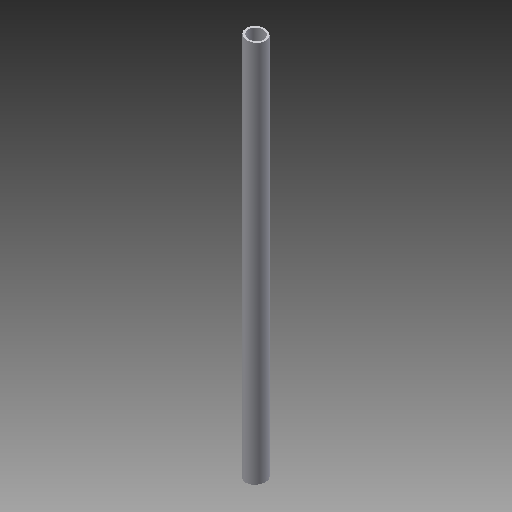
# Autodesk Inventor part: Rura_poprzeczna_ergosiedziska
Saved by Autodesk Inventor 2017 (Build 210142000, 142)
## iProperties
Created: 2015-11-20
Part Number: Rura_poprzeczna_ergosiedziska
Material: Aluminium AW-7020
Document SubType Name: Modelowanie
Designer: graaapsik
Density: 2.78 g/cm^3
Appearance: Aluminium AW-7020
Sheet Metal Rule: Default
Mass: 125.214 g
Surface Area: 452.681 cm^2
Volume: 45.041 cm^3
Author: graaapsik
Autodesk Inventor part; units mm, degrees
ref_plane "YZ Plane" through (0, 0, 0) normal (1, 0, 0) x (0, 1, 0)
ref_plane "XZ Plane" through (0, 0, 0) normal (0, 1, 0) x (-1, 0, 0)
ref_plane "XY Plane" through (0, 0, 0) normal (0, 0, 1) x (1, 0, 0)
sketch "Szkic1" plane through (0, 0, 0) normal (0, 1, 0) x (-1, 0, 0)
  circle A0 centre (0, 0) radius 10
  dimension "d0" = 20
  constraints: 1 centre point, 1 coincident
  measures "d0" diameter of A0
extrude "Wyciągnięcie proste1" add sketch "Szkic1" along normal blind 400
shell "Skorupa1" thickness 2 removed faces 2 at (1.182, 0, 3.1167) at (1.182, 400, 3.1167)
sketch "Szkic2" plane through (0, 0, 0) normal (0, 0, 1) x (1, 0, 0)
  line L0 (-10, 0) -> (10, 0) construction
  line L1 (-10, 0) -> (10, 0)
  line L2 (22.37, 2.832) -> (-10, 0)
  line L3 (10, 0) -> (22.37, 2.832)
  line L4 (10, 400) -> (-10, 400) construction
  line L5 (10, 0) -> (10, 400) construction
  line L6 (-10, 400) -> (10, 400)
  line L7 (10, 400) -> (10, 398.2502)
  line L8 (10, 398.2502) -> (-10, 400)
  point P0 (0, 0)
  dimension "d4" = 5
  dimension "d7" = 5
  constraints: 12 end point, 2 point on line, 1 collinear
  measures "d4" angle of L1 L2
  measures "d7" angle of L8 L6
extrude "Wyciągnięcie proste3" cut sketch "Szkic2" along normal mid plane 32
equation "\"PromieńGięcia\" = Grubość"
equation "\"SzerokośćGięciaPodcięcia\" = Grubość"
equation "\"GłębokośćGięciaPodcięcia\" = 0.5 * Grubość"
equation "\"RozmiarPodcięciaNarożnika\" = 4 * Grubość"
equation "\"MinimalnaPozostałość\" = 2 * Grubość"
equation "\"PromieńPrzejścia\" = PromieńGięcia"
equation "\"Rozmiar_promienia_Jacobiego\" = Grubość"
equation "\"Wielk_odstępu\" = Grubość"
equation "\"Grubość\" = 0.5"
